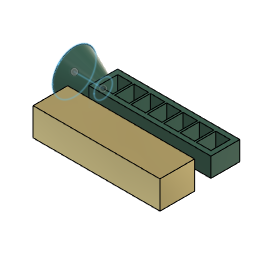
ADHPillBox v2 (Autodesk Fusion 360 design; units mm, degrees)
Autodesk Fusion 360 part; units mm, degrees
note: some values were not read from the file. Set by a fixed rule: which face or edge a step refers to.
sketch "Sketch1" plane through (0, 0, 0) normal (0, 0, 1) x (1, 0, 0)
  line L0 (33.9081, 20.4446) -> (150.9081, 20.4446)
  line L1 (150.9081, 20.4446) -> (150.9081, 40.4446)
  line L2 (150.9081, 40.4446) -> (33.9081, 40.4446)
  line L3 (33.9081, 40.4446) -> (33.9081, 20.4446)
  line L4 (28.9081, 20.4446) -> (28.9081, 15.4446)
  line L5 (28.9081, 15.4446) -> (155.9081, 15.4446)
  line L6 (155.9081, 15.4446) -> (155.9081, 45.4446)
  line L7 (155.9081, 45.4446) -> (28.9081, 45.4446)
  line L8 (28.9081, 45.4446) -> (28.9081, 15.4446)
  line L9 (33.9081, 40.4446) -> (48.9081, 40.4446)
  line L10 (48.9081, 40.4446) -> (50.9081, 40.4446)
  line L11 (50.9081, 40.4446) -> (50.9081, 20.4446)
  line L12 (50.9081, 20.4446) -> (48.9081, 20.4446)
  line L13 (48.9081, 20.4446) -> (48.9081, 40.4446)
  line L14 (50.9081, 40.4446) -> (65.9081, 40.4446)
  line L15 (65.9081, 40.4446) -> (67.9081, 40.4446)
  line L16 (67.9081, 40.4446) -> (67.9081, 20.4446)
  line L17 (67.9081, 20.4446) -> (65.9081, 20.4446)
  line L18 (65.9081, 20.4446) -> (65.9081, 40.4446)
  line L19 (67.9081, 40.4446) -> (82.9081, 40.4446)
  line L20 (82.9081, 40.4446) -> (84.9081, 40.4446)
  line L21 (84.9081, 40.4446) -> (84.9081, 20.4446)
  line L22 (84.9081, 20.4446) -> (82.9081, 20.4446)
  line L23 (82.9081, 20.4446) -> (82.9081, 40.4446)
  line L24 (99.9081, 40.4446) -> (101.9081, 40.4446)
  line L25 (101.9081, 40.4446) -> (101.9081, 20.4446)
  line L26 (101.9081, 20.4446) -> (99.9081, 20.4446)
  line L27 (99.9081, 20.4446) -> (99.9081, 40.4446)
  line L28 (116.9081, 40.4446) -> (118.9081, 40.4446)
  line L29 (118.9081, 40.4446) -> (118.9081, 20.4446)
  line L30 (118.9081, 20.4446) -> (116.9081, 20.4446)
  line L31 (116.9081, 20.4446) -> (116.9081, 40.4446)
  line L32 (133.9081, 40.4446) -> (135.9081, 40.4446)
  line L33 (135.9081, 40.4446) -> (135.9081, 20.4446)
  line L34 (135.9081, 20.4446) -> (133.9081, 20.4446)
  line L35 (133.9081, 20.4446) -> (133.9081, 40.4446)
  dimension "d1" = 117
  dimension "d2" = 20
  dimension "d3" = 5
  dimension "d4" = 5
  dimension "d5" = 127
  dimension "d6" = 30
  dimension "d7" = 15
  dimension "d8" = 2
  dimension "d9" = 15
  dimension "d10" = 2
  dimension "d11" = 15
  dimension "d12" = 2
  dimension "d13" = 15
  dimension "d14" = 2
  dimension "d15" = 15
  dimension "d16" = 2
  dimension "d17" = 15
  dimension "d18" = 2
  constraint horizontal L0
  constraint vertical L1
  constraint horizontal L2
  constraint vertical L3
  constraint horizontal L5
  constraint vertical L6
  constraint horizontal L7
  constraint vertical L8
  constraint perpendicular L3 L9
  constraint horizontal L10
  constraint vertical L11
  constraint horizontal L12
  constraint vertical L13
  constraint perpendicular L11 L14
  constraint horizontal L15
  constraint vertical L16
  constraint horizontal L17
  constraint vertical L18
  constraint perpendicular L16 L19
  constraint horizontal L20
  constraint vertical L21
  constraint horizontal L22
  constraint vertical L23
  constraint horizontal L24
  constraint vertical L25
  constraint horizontal L26
  constraint vertical L27
  constraint horizontal L28
  constraint vertical L29
  constraint horizontal L30
  constraint vertical L31
  constraint horizontal L32
  constraint vertical L33
  constraint horizontal L34
  constraint vertical L35
  measures "d1" distance of L0.start L0.end
  measures "d2" distance of L0.start L2.end
  measures "d3" distance of L0.start L4.start
  measures "d4" distance of L4.start L4.end
  measures "d5" distance of L4.end L5.end
  measures "d6" distance of L4.end L7.end
  measures "d7" distance of L2.end L9.end
  measures "d8" distance of L9.end L10.end
  measures "d9" distance of L10.end L14.end
  measures "d10" distance of L14.end L15.end
  measures "d11" distance of L15.end L19.end
  measures "d12" distance of L19.end L20.end
  measures "d13" distance of L20.end L24.start
  measures "d14" distance of L24.start L24.end
  measures "d15" distance of L24.end L28.start
  measures "d16" distance of L28.start L28.end
  measures "d17" distance of L28.end L32.start
  measures "d18" distance of L32.start L32.end
extrude "Extrude1" add sketch "Sketch1" along normal blind 15 contours L0 L2 L10 L11 L12 L13 | L0 L2 L15 L16 L17 L18 | L0 L2 L20 L21 L22 L23 | L0 L2 L24 L25 L26 L27 | L0 L2 L28 L29 L30 L31 | L0 L2 L32 L33 L34 L35 | L4 L5 L6 L7 L8 makes body 1
extrude "Extrude2" add sketch "Sketch1" against normal blind 2 contours L0 L2 L3 L9 L13 | L0 L2 L10 L11 L12 L13 | L0 L2 L11 L14 L18 | L0 L2 L15 L16 L17 L18 | L0 L2 L16 L19 L23 | L0 L2 L20 L21 L22 L23 | L0 L2 L21 L27 | L0 L2 L24 L25 L26 L27 | L0 L2 L25 L31 | L0 L2 L28 L29 L30 L31 | L0 L2 L29 L35 | L0 L2 L32 L33 L34 L35 | L0 L1 L2 L33 | L4 L5 L6 L7 L8 bodies 1
move_body "Move1" bodies 1 to x (1, 0, 0) y (0, 1, 0) z (0, 0, 1) at (0, 0, 2)
sketch "Sketch2" plane through (0, 0, 0) normal (0, 0, -1) x (1, 0, 0)
  line L0 (28.9081, -15.4446) -> (28.9081, -45.4446)
  line L1 (28.9081, -45.4446) -> (155.9081, -45.4446)
  line L2 (155.9081, -45.4446) -> (155.9081, -15.4446)
  line L3 (155.9081, -15.4446) -> (28.9081, -15.4446)
  line L4 (150.9081, -40.4446, -2) -> (135.9081, -40.4446, -2)
  line L5 (135.9081, -40.4446, -2) -> (135.9081, -20.4446, -2)
  line L6 (135.9081, -20.4446, -2) -> (150.9081, -20.4446, -2)
  line L7 (150.9081, -20.4446, -2) -> (150.9081, -40.4446, -2)
  line L8 (133.9081, -40.4446, -2) -> (118.9081, -40.4446, -2)
  line L9 (118.9081, -40.4446, -2) -> (118.9081, -20.4446, -2)
  line L10 (118.9081, -20.4446, -2) -> (133.9081, -20.4446, -2)
  line L11 (133.9081, -20.4446, -2) -> (133.9081, -40.4446, -2)
  line L12 (116.9081, -40.4446, -2) -> (101.9081, -40.4446, -2)
  line L13 (101.9081, -40.4446, -2) -> (101.9081, -20.4446, -2)
  line L14 (101.9081, -20.4446, -2) -> (116.9081, -20.4446, -2)
  line L15 (116.9081, -20.4446, -2) -> (116.9081, -40.4446, -2)
  line L16 (99.9081, -40.4446, -2) -> (84.9081, -40.4446, -2)
  line L17 (84.9081, -40.4446, -2) -> (84.9081, -20.4446, -2)
  line L18 (84.9081, -20.4446, -2) -> (99.9081, -20.4446, -2)
  line L19 (99.9081, -20.4446, -2) -> (99.9081, -40.4446, -2)
  line L20 (82.9081, -40.4446, -2) -> (67.9081, -40.4446, -2)
  line L21 (67.9081, -40.4446, -2) -> (67.9081, -20.4446, -2)
  line L22 (67.9081, -20.4446, -2) -> (82.9081, -20.4446, -2)
  line L23 (82.9081, -20.4446, -2) -> (82.9081, -40.4446, -2)
  line L24 (65.9081, -40.4446, -2) -> (50.9081, -40.4446, -2)
  line L25 (50.9081, -40.4446, -2) -> (50.9081, -20.4446, -2)
  line L26 (50.9081, -20.4446, -2) -> (65.9081, -20.4446, -2)
  line L27 (65.9081, -20.4446, -2) -> (65.9081, -40.4446, -2)
  line L28 (48.9081, -40.4446, -2) -> (33.9081, -40.4446, -2)
  line L29 (33.9081, -40.4446, -2) -> (33.9081, -20.4446, -2)
  line L30 (33.9081, -20.4446, -2) -> (48.9081, -20.4446, -2)
  line L31 (48.9081, -20.4446, -2) -> (48.9081, -40.4446, -2)
  point P0 (150.9081, -40.4446)
  point P1 (135.9081, -20.4446)
  point P2 (133.9081, -40.4446)
  point P3 (118.9081, -20.4446)
  point P4 (116.9081, -40.4446)
  point P5 (101.9081, -20.4446)
  point P6 (99.9081, -40.4446)
  point P7 (84.9081, -20.4446)
  point P8 (82.9081, -40.4446)
  point P9 (67.9081, -20.4446)
  point P10 (65.9081, -40.4446)
  point P11 (50.9081, -20.4446)
  point P12 (48.9081, -40.4446)
  point P13 (33.9081, -20.4446)
sketch "Sketch3" plane through (0, 0, 2) normal (0, 0, -1) x (1, 0, 0)
sketch "Sketch4" plane through (0, 0, 2) normal (0, 0, -1) x (1, 0, 0)
  circle A0 centre (41.4081, -30.4446) radius 1.5
  circle A1 centre (58.4081, -30.4446) radius 1.5
  circle A2 centre (75.4081, -30.4446) radius 1.5
  circle A3 centre (92.4081, -30.4446) radius 1.5
  circle A4 centre (109.4081, -30.4446) radius 1.5
  circle A5 centre (126.4081, -30.4446) radius 1.5
  circle A6 centre (143.4081, -30.4446) radius 1.5
  dimension "d23" = 3
  dimension "d24" = 3
  dimension "d25" = 3
  dimension "d26" = 3
  dimension "d27" = 3
  dimension "d28" = 3
  dimension "d29" = 3
  measures "d23" diameter of A0
  measures "d24" diameter of A1
  measures "d25" diameter of A2
  measures "d26" diameter of A3
  measures "d27" diameter of A4
  measures "d28" diameter of A5
  measures "d29" diameter of A6
extrude "Extrude3" add sketch "Sketch2" along normal blind 3 bodies 1
extrude "Extrude4" cut sketch "Sketch4" along normal blind 5 bodies 1
extrude "Extrude5" add sketch "Sketch4" along normal blind 2.9 bodies 1
copy_body "CopyPasteBodies1" bodies 1 makes body 2
move_body "Move2" bodies 2 to x (1, 0, 0) y (0, 1, 0) z (0, 0, 1) at (0, 0, 0)
move_body "Move3" bodies 2 to x (1, 0, 0) y (0, 1, 0) z (0, 0, 1) at (-145, 0, 0)
move_body "Move4" bodies 2 to x (1, 0, 0) y (0, -1, 0) z (0, 0, -1) at (0, 60.8891, 14)
sketch "Sketch5" plane through (-116.0919, 0, 0) normal (-1, 0, 0) x (0, -1, 0)
  line L0 (-45.4446, 17) -> (-45.4446, -3)
  line L1 (-45.4446, -3) -> (-15.4446, -3)
  line L2 (-15.4446, -3) -> (-15.4446, 17)
  line L3 (-15.4446, 17) -> (-45.4446, 17)
  line L4 (-45.4446, 17) -> (-15.4446, 17)
  line L5 (-15.4446, 17) -> (-15.4446, -3)
  line L6 (-15.4446, -3) -> (-45.4446, -3)
  line L7 (-45.4446, -3) -> (-45.4446, 17)
  line L8 (-46.4446, 18) -> (-14.4446, 18)
  line L9 (-14.4446, 18) -> (-14.4446, -4)
  line L10 (-14.4446, -4) -> (-46.4446, -4)
  line L11 (-46.4446, -4) -> (-46.4446, 18)
  constraint horizontal L4
  constraint vertical L5
  constraint horizontal L6
  constraint vertical L7
  constraint coincident L1.end L2.start
  constraint coincident L0.start L3.end
  constraint horizontal L8
  constraint vertical L9
  constraint horizontal L10
  constraint vertical L11
extrude "Extrude6" add 7 faces at (-106.0919, 27.1112, 12) (-89.0919, 27.1112, 12) (-72.0919, 27.1112, 12) (-55.0919, 27.1112, 12) (-33.0919, 33.7779, 12) (-21.0919, 27.1112, 12) (-4.0919, 27.1112, 12) along direction (0, 0, -1) blind 15 on bodies 2 bodies 2
extrude "Extrude7" add 1 faces at (-52.5707, 19.945, 17) along direction (0, 0, 1) blind 6 on bodies 2 bodies 2
extrude "Extrude8" add 1 faces at (-31.4253, 45.4446, 5.6667) along direction (0, 1, 0) blind 3 on bodies 2 bodies 2
extrude "Extrude9" add 1 faces at (-73.7586, 26.4446, -3) along direction (0, 0, -1) blind 3 on bodies 2 bodies 2
extrude "Extrude10" add 1 faces at (-73.7586, 15.4446, 3.6667) along direction (0, -1, 0) blind 3 on bodies 2 bodies 2
extrude "Extrude11" cut sketch "Sketch5" against normal blind 127 contours L0 L1 L2 L3 L4 L5 L6 L7 | L8 L9 L10 L11 bodies 2
sketch "Sketch6" plane through (10.9081, 0, 0) normal (1, 0, 0) x (0, 1, 0)
  line L0 (14.4446, -4) -> (14.4446, 18)
  line L1 (14.4446, 18) -> (46.4446, 18)
  line L2 (46.4446, 18) -> (46.4446, -4)
  line L3 (46.4446, -4) -> (14.4446, -4)
  line L4 (12.4446, -6) -> (48.4446, -6)
  line L5 (48.4446, -6) -> (48.4446, 23)
  line L6 (48.4446, 23) -> (12.4446, 23)
  line L7 (12.4446, 23) -> (12.4446, -6)
  line L8 (46.4446, -4) -> (14.4446, -4)
  line L9 (14.4446, -4) -> (14.4446, 18)
  line L10 (14.4446, 18) -> (46.4446, 18)
  line L11 (46.4446, 18) -> (46.4446, -4)
  constraint horizontal L8
  constraint vertical L9
  constraint horizontal L10
  constraint vertical L11
  constraint coincident L0.end L1.start
  constraint coincident L2.end L3.start
extrude "Extrude12" add sketch "Sketch6" along normal blind 3 contours L0 L1 L2 L3 L8 L9 L10 L11 | L4 L5 L6 L7 bodies 2
extrude "Extrude13" add 1 faces at (13.9081, 24.4446, 13.3333) along direction (1, 0, 0) blind 2 on bodies 2 bodies 2
extrude "Extrude14" cut 1 faces at (10.9081, 25.1112, 3.3333) along direction (1, 0, 0) blind 1 on bodies 2 bodies 2
sketch "Sketch7" plane through (0, 0, 18) normal (0, 0, -1) x (1, 0, 0)
  circle A0 centre (-35.5919, -30.4446) radius 1.5
  circle A1 centre (-103.5919, -30.4446) radius 1.5
  circle A2 centre (-52.5919, -30.4446) radius 1.5
  circle A3 centre (-18.5919, -30.4446) radius 1.5
  circle A4 centre (-86.5919, -30.4446) radius 1.5
  circle A5 centre (-69.5919, -30.4446) radius 1.5
  circle A6 centre (-1.5919, -30.4446) radius 1.5
  line L0 (-116.0919, -14.4446) -> (-116.0919, -46.4446)
  line L1 (-116.0919, -46.4446) -> (11.9081, -46.4446)
  line L2 (11.9081, -46.4446) -> (11.9081, -14.4446)
  line L3 (11.9081, -14.4446) -> (-116.0919, -14.4446)
  circle A7 centre (-1.5919, -30.4446) radius 1.5
  circle A8 centre (-18.5919, -30.4446) radius 1.5
  circle A9 centre (-35.5919, -30.4446) radius 1.5
  circle A10 centre (-52.5919, -30.4446) radius 1.5
  circle A11 centre (-69.5919, -30.4446) radius 1.5
  circle A12 centre (-86.5919, -30.4446) radius 1.5
  circle A13 centre (-103.5919, -30.4446) radius 1.5
  constraint concentric A6 A7
  constraint concentric A3 A8
  constraint concentric A0 A9
  constraint concentric A2 A10
  constraint concentric A5 A11
  constraint concentric A4 A12
  constraint concentric A1 A13
extrude "Extrude15" add sketch "Sketch7" against normal blind 2.9 contours A0 A9 | A1 A13 | A2 A10 | A3 A8 | A4 A12 | A5 A11 | A6 A7 bodies 2
move_body "Move5" bodies 1 to x (1, 0, 0) y (0, 1, 0) z (0, 0, 1) at (-140, 50, 0)
sketch "Sketch8" plane through (-111.0919, 0, 0) normal (-1, 0, 0) x (0, -1, 0)
  line L0 (-65.4446, -3) -> (-65.4446, 17)
  line L1 (-65.4446, 17) -> (-95.4446, 17)
  line L2 (-95.4446, 17) -> (-95.4446, -3)
  line L3 (-95.4446, -3) -> (-65.4446, -3)
  circle A0 centre (-80.4446, 7) radius 9.5
  line L4 (-80.4446, 7, 0) -> (-80.4446, 7, 30)
  circle A1 through (-57.9446, 7, 30) (-91.6946, 26.4856, 30) (-91.6946, -12.4856, 30)
  dimension "d60" = 19
  dimension "d61" = 30
  dimension "d62" = 45
  measures "d60" diameter of A0
sketch "Sketch9" plane through (-111.0919, 0, 0) normal (-1, 0, 0) x (0, -1, 0)
  circle A0 centre (-80.4446, 7) radius 9.5
  circle A1 through (-57.9446, 7, 30) (-91.6946, 26.4856, 30) (-91.6946, -12.4856, 30)
  point P0 (-80.4446, 7)
  point P1 (-80.4446, 7)
loft "Loft1" add profiles "Sketch9", "Sketch9" section 1 contours A1 in plane through (-141.0919, 0, 0) normal (-1, 0, 0) section 2 bodies 1
sketch "Sketch10" plane through (0, 0, 23) normal (0, 0, 1) x (-1, 0, 0)
  circle A0 centre (35.5919, -30.4446) radius 1.5
  circle A1 centre (103.5919, -30.4446) radius 1.5
  circle A2 centre (52.5919, -30.4446) radius 1.5
  circle A3 centre (18.5919, -30.4446) radius 1.5
  circle A4 centre (86.5919, -30.4446) radius 1.5
  circle A5 centre (69.5919, -30.4446) radius 1.5
  circle A6 centre (1.5919, -30.4446) radius 1.5
  line L0 (116.0919, -48.4446) -> (116.0919, -12.4446)
  line L1 (116.0919, -12.4446) -> (-15.9081, -12.4446)
  line L2 (-15.9081, -12.4446) -> (-15.9081, -48.4446)
  line L3 (-15.9081, -48.4446) -> (116.0919, -48.4446)
  circle A7 centre (1.5919, -30.4446) radius 1.5
  circle A8 centre (18.5919, -30.4446) radius 1.5
  circle A9 centre (35.5919, -30.4446) radius 1.5
  circle A10 centre (52.5919, -30.4446) radius 1.5
  circle A11 centre (69.5919, -30.4446) radius 1.5
  circle A12 centre (86.5919, -30.4446) radius 1.5
  circle A13 centre (103.5919, -30.4446) radius 1.5
  constraint concentric A6 A7
  constraint concentric A3 A8
  constraint concentric A0 A9
  constraint concentric A2 A10
  constraint concentric A5 A11
  constraint concentric A4 A12
  constraint concentric A1 A13
extrude "Extrude16" cut sketch "Sketch10" against normal blind 5 contours A0 A9 | A1 A13 | A2 A10 | A3 A8 | A4 A12 | A5 A11 | A6 A7 bodies 2
extrude "Extrude17" add sketch "Sketch10" against normal blind 2.9 contours A0 A9 | A1 A13 | A2 A10 | A3 A8 | A4 A12 | A5 A11 | A6 A7 bodies 2
equation "d1 = ( 7 * 15 ) * 1 mm + ( 6 * 2 ) * 1 mm"
